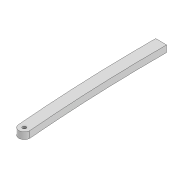
# Autodesk Inventor part: Part_8_p2
Saved by Autodesk Inventor 2022 (Build 260153000, 153)
## iProperties
Created: 2022-04-22
Part Number: Part_8_p2
Material: Generic
Document SubType Name: Modeling
Designer: dell
Density: 1 g/cm^3
Appearance: Default
Mass: 3.16724 g
Surface Area: 27.4249 cm^2
Volume: 3.16724 cm^3
Author: dell
Autodesk Inventor part; units mm, degrees
ref_plane "YZ Plane" through (0, 0, 0) normal (1, 0, 0) x (0, 1, 0)
ref_plane "XZ Plane" through (0, 0, 0) normal (0, 1, 0) x (-1, 0, 0)
ref_plane "XY Plane" through (0, 0, 0) normal (0, 0, 1) x (1, 0, 0)
sketch "Sketch1" plane through (0, 0, 0) normal (0, 1, 0) x (-1, 0, 0)
  line L0 (0, 0) -> (0, -253.429) construction
  line L1 (5, 0) -> (5, -253.429)
  line L2 (-5, -253.429) -> (-5, 0)
  arc A0 (5, 0) -> (-5, 0) centre (0, 0) ccw
  arc A1 (-5, -253.429) -> (5, -253.429) centre (0, -253.429) ccw
  circle A2 centre (0, 0) radius 1.65
  circle A3 centre (0, -253.429) radius 1.65
  arc A4 (5, -253.429) -> (5, 0) centre (-1489.6382, -126.7145) ccw
  arc A5 (-5, -253.429) -> (-5, 0) centre (-1499.6382, -126.7145) ccw
  point P0 (0, -126.7145)
  dimension "d0" = 3.3
  dimension "d1" = 3.3
  dimension "d2" = 10
  dimension "d3" = 253.429
  dimension "d16" = 1500
  dimension "d17" = 1500
  constraints: 8 end point, 8 point on circle, 6 centre point, 4 tangent, 2 coincident, 1 midpoint, 1 parallel, 1 vertical
  measures "d0" diameter of A2
  measures "d1" diameter of A3
  measures "d2" distance between parallel lines of L2 L1
  measures "d3" distance of L0.end L0.start
  measures "d16" radius of A4
  measures "d17" radius of A5
extrude "Extrusion1" add sketch "Sketch1" along normal blind 6 contours A4 L1 | L1 A1 A5 A0
sketch "Sketch2" plane through (0, 6, 0) normal (0, 1, 0) x (1, 0, 0)
  line L0 (-27.9396, 271.9091) -> (26.8888, 271.9091)
  line L1 (26.8888, 271.9091) -> (26.8888, 130.022)
  line L2 (26.8888, 130.022) -> (-27.9396, 130.022)
  line L3 (-27.9396, 130.022) -> (-27.9396, 271.9091)
  line L4 (-79.0634, 296.7301) -> (75.0489, 296.7301)
  line L5 (75.0489, 296.7301) -> (75.0489, -47.4295)
  line L6 (75.0489, -47.4295) -> (-79.0634, -47.4295)
  line L7 (-79.0634, -47.4295) -> (-79.0634, 296.7301)
  point P0 (0, 0)
  constraints: 16 end point, 4 parallel, 2 horizontal, 2 perpendicular
extrude "Extrusion2" cut sketch "Sketch2" against normal blind 10 contours L0 L1 L2 L3
body "Solid1"
